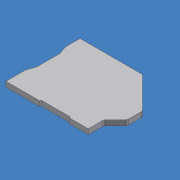
# Autodesk Inventor part: 745-300
Saved by Autodesk Inventor 2012 (Build 160160000, 160)
## iProperties
Company: Team 801
Created: 2007-09-01
Part Number: 745-300
Catalog Web Link: www.team801.org
Description: 745-300 - END PLATE SNAP FIT TYPE 1.5 MM / 0.059 IN THICK
Document SubType Name: Modeling
Designer: Jeffrey M
Mass: 0.921082 g
Surface Area: 13.0584 cm^2
Volume: 0.921082 cm^3
Density: 1 g/cm^3
Material: Default
NB: 745-300
NN: 745-300
NT: END PLATE SNAP FIT TYPE 1.5 MM / 0.059 IN THICK
NBSYN: $BESTNR.
LINA: 745-300
BESTNR: 745-300
HOEHE: 23.00
BREITE: 1.60
TIEFE: 29.10
FARBE: grau
GEWICHT: 0.670
EAN: 4017332608152
RGB: 0.67,0.67,0.67,0
KT: DUMMY
PSOL_IDENT_0: {\\partserver001.servicenet\dplatte\cadenas\23d-libs\wago\pg04\serie745\0745-0300_0999-0962.prj},149
PSOL_IDENT_1: {VTYP=3D},{NB=745-300},{LINA=745-300},{NN=745-300},{DATE=24.01.2007 11:36:55},{GEOMDATE=13.06.2006}
PSOL_IDENT_2: ,{VERSION=},{LINEID=160},{LINESUBID=-1},{WBVAR=}  {NB=745-300},{LINA=745-300},{KT=DUMMY},{BESTNR=745
PSOL_IDENT_3: -300},{HOEHE=23.00},{BREITE=1.60},{TIEFE=29.10},{FARBE=grau},{GEWICHT=0.670},{EAN=4017332608152},{RG
PSOL_IDENT_4: B=0.67,0.67,0.67,0}
Title: 745-300
Author: Jeffrey M
Autodesk Inventor part; units mm, degrees
ref_plane "YZ Plane" through (0, 0, 0) normal (1, 0, 0) x (0, 1, 0)
ref_plane "XZ Plane" through (0, 0, 0) normal (0, 1, 0) x (-1, 0, 0)
ref_plane "XY Plane" through (0, 0, 0) normal (0, 0, 1) x (1, 0, 0)
sketch "Skizze_1" plane through (0, 0, 0) normal (0, 0, 1) x (1, 0, 0)
  line L0 (-20.9, 0) -> (-10.5, 0)
  line L1 (-10.5, 0) -> (-10.5, 0.4)
  line L2 (-10.5, 0.4) -> (-1.5, 0.4)
  line L3 (-1.5, 0.4) -> (-1.5, 0)
  line L4 (-1.5, 0) -> (4.4, 0)
  line L5 (4.4, 0) -> (4.4, 4.3858)
  arc A0 (4.6929, 5.0929) -> (4.4, 4.3858) centre (5.4, 4.3858) ccw
  line L6 (4.6929, 5.0929) -> (7.7071, 8.1071)
  arc A1 (7.7071, 8.1071) -> (8, 8.8142) centre (7, 8.8142) ccw
  line L7 (8, 8.8142) -> (8, 12.6858)
  arc A2 (8, 12.6858) -> (7.7071, 13.3929) centre (7, 12.6858) ccw
  line L8 (7.7071, 13.3929) -> (-1.4071, 22.5071)
  arc A3 (-1.4071, 22.5071) -> (-2.1142, 22.8) centre (-2.1142, 21.8) ccw
  line L9 (-2.1142, 22.8) -> (-20.9, 22.8)
  line L10 (-20.9, 22.8) -> (-20.9, 18.2727)
  line L11 (-20.9, 18.2727) -> (-20, 15.8)
  line L12 (-20, 15.8) -> (-20, 8.5)
  line L13 (-20, 8.5) -> (-20.9, 6.0273)
  line L14 (-20.9, 6.0273) -> (-20.9, 0)
  constraints: 30 end point, 8 point on circle, 4 centre point
extrude "Extrusion1" add sketch "Skizze_1" along normal blind 1.6
body "Solid1"
